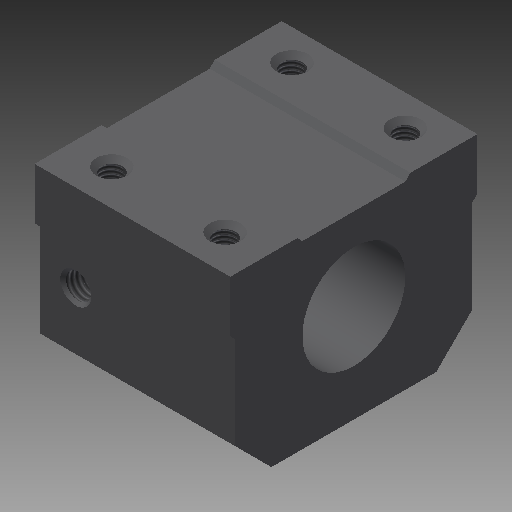
# Autodesk Inventor part: BNT 2010-2.6 Nut
Saved by Autodesk Inventor 2018 (Build 220112000, 112)
## iProperties
Category: PARTsolutions
Company: THK
Created: 2017-05-30
Part Number: BNT 2010-2.6 Nut
Catalog Web Link: www.cadenas.de
Description: BNT Nut-
Vendor: THK
Document SubType Name: Modeling
Designer: psAdmin
Manufacturer: THK
Mass: 82.4787 g
Surface Area: 175.198 cm^2
Volume: 82.4787 cm^3
Density: 1 g/cm^3
Material: Generic
Appearance: PSOLRGB-192-192-192
PSOL_IDENT_0: {$CADENAS_DATA\23d-libs\thk\fed_screw\ball_screw\ball_screw\standard_lead_rbs\bnt\bnt_nut.prj},176 {
PSOL_IDENT_1: VTYP=3D},{NB=BNT 2010-2.6 Nut},{LINA=BNT 2010-2.6 Nut},{NN=BNT Nut},{DATE=16.05.2017 06:09:49},{GEOM
PSOL_IDENT_2: DATE=23.11.2007 13:11:00},{VERSION=},{LINEID=290},{LINESUBID=-1},{WBVAR=}  {NB=BNT 2010-2.6 Nut},{LI
PSOL_IDENT_3: NA=BNT 2010-2.6 Nut},{KT=DUMMY},{MN=BNT 2010-2.6},{L=58.000},{EL=2102.000},{W=48.000},{F=18.000},{B=
PSOL_IDENT_4: 35.000},{C=35.000},{W1=24.000},{T=9.000},{M=46.000},{NDM=6.000},{KDM=4.917},{SL=10.000},{N1=10.000},
PSOL_IDENT_5: {N2=2.000},{A=6.000},{M1=41.400},{X1=1.440},{X2=20.700},{R1=10.170},{X3=4.560},{ANG=47.0},{DK=4.000}
PSOL_IDENT_6: ,{Y=1.770},{X4=0.300},{SD=20},{SL2=10.000},{Y2=14.560}
NN: BNT Nut
NB: BNT 2010-2.6 Nut
NBSYN: $MN. Nut
LINA: BNT 2010-2.6 Nut
MN: BNT 2010-2.6
L: 58.000
EL: 2102.000
W: 48.000
F: 18.000
B: 35.000
C: 35.000
W1: 24.000
T: 9.000
M: 46.000
NDM: 6.000
KDM: 4.917
SL: 10.000
N1: 10.000
N2: 2.000
A: 6.000
M1: 41.400
X1: 1.440
X2: 20.700
R1: 10.170
X3: 4.560
ANG: 47.0
DK: 4.000
Y: 1.770
X4: 0.300
SD: 20
SL2: 10.000
Y2: 14.560
SUPPLIER: THK
ARTICLENO: BNT 2010-2.6 Nut
BOMINFO: BNT 2010-2.6 Nut
CREATOR: CADENAS GmbH
Title: BNT 2010-2.6 Nut
Author: Cadenas PARTsolutions
Autodesk Inventor part; units mm, degrees
ref_plane "YZ Plane" through (0, 0, 0) normal (1, 0, 0) x (0, 1, 0)
ref_plane "XZ Plane" through (0, 0, 0) normal (0, 1, 0) x (-1, 0, 0)
ref_plane "XY Plane" through (0, 0, 0) normal (0, 0, 1) x (1, 0, 0)
sketch "Sketch_1" plane through (0, 0, 0) normal (1, 0, 0) x (0, 1, 0)
  line L0 (17, 24) -> (7, 24)
  line L1 (7, 24) -> (6, 23)
  line L2 (6, 23) -> (-12, 23)
  line L3 (-19, 16) -> (-19, -16)
  line L4 (-12, -23) -> (6, -23)
  line L5 (6, -23) -> (7, -24)
  line L6 (7, -24) -> (17, -24)
  line L7 (17, -24) -> (17, -11)
  line L8 (17, -11) -> (16, -10)
  line L9 (16, -10) -> (16, 10)
  line L10 (16, 10) -> (17, 11)
  line L11 (17, 11) -> (17, 24)
  circle A0 centre (0, 0) radius 10
  line L12 (16, 0) -> (0, 0) construction
  line L13 (-12, -23) -> (-19, -16)
  line L14 (-12, 23) -> (-19, 16)
  line L15 (0, 0) -> (-19, 0) construction
  line L16 (6, 23) -> (6, -23) construction
  dimension "d39" = 20
  dimension "d41" = 46
  dimension "d43" = 23
  dimension "d45" = 1
  dimension "d46" = 48
  dimension "d47" = 1
  dimension "d48" = 36
  dimension "d49" = 10
  dimension "d50" = 10
  dimension "d51" = 20
  dimension "d52" = 13
  dimension "d53" = 13
  dimension "d54" = 32
  dimension "d55" = 16
  dimension "d56" = 135
  dimension "d57" = 18
  dimension "d58" = 18
  constraints: 34 end point, 2 coincident, 2 horizontal, 2 midpoint, 2 parallel, 2 vertical, 1 centre point, 1 collinear, 1 perpendicular, 1 other
  measures "d39" diameter of A0
  measures "d41" distance between parallel lines of L4 L2
  measures "d43" distance from line of L2 L12.end
  measures "d45" distance between parallel lines of L9 L7
  measures "d46" distance between parallel lines of L6 L0
  measures "d47" distance between parallel lines of L4 L6
  measures "d48" distance between parallel lines of L7 L3
  measures "d49" distance of L0.start L0.end
  measures "d50" distance of L5.end L6.end
  measures "d51" distance of L8.end L9.end
  measures "d52" distance of L10.end L0.start
  measures "d53" distance of L6.end L7.end
  measures "d54" distance of L3.start L3.end
  measures "d55" distance from line of L9 L12.end
  measures "d56" angle of L0 L1
  measures "d57" distance of L4.start L4.end
  measures "d58" distance of L1.end L2.end
extrude "Extrusion1" add sketch "Sketch_1" along normal blind 38
sketch "Sketch_2" plane through (29, 0, 0) normal (0.6819984, 0, 0.7313537) x (0.7313537, 0, -0.6819984)
  line L0 (-29, -24.55) -> (-4.4539, -24.55)
  arc A0 (-4.4539, -24.55) -> (4.4539, -24.55) centre (0, -23.4) ccw
  line L1 (4.4539, -24.55) -> (29, -24.55)
  line L2 (29, -24.55) -> (29, -23.4)
  line L3 (29, -23.4) -> (-29, -23.4)
  line L4 (-29, -23.4) -> (-29, -24.55)
  dimension "d33" = 58
  dimension "d34" = 1.15
  dimension "d35" = 24.5461
  dimension "d36" = 4.6
  dimension "d37" = 24.5461
  dimension "d38" = 1.15
  constraints: 10 end point, 2 point on circle, 1 centre point, 1 midpoint, 1 perpendicular
  measures "d33" distance of L2.end L3.end
  measures "d34" distance of L1.end L2.end
  measures "d35" distance of L1.start L1.end
  measures "d36" radius of A0
  measures "d37" distance of L0.start L0.end
  measures "d38" distance of L3.end L0.start
extrude "Extrusion2" [suppressed]
sketch "Sketch_3" plane through (0, -23.4, 0) normal (0, 1, 0) x (1, 0, 0)
  line L0 (-29, -58) -> (87, -58)
  line L1 (87, -58) -> (87, 58)
  line L2 (87, 58) -> (-29, 58)
  line L3 (-29, 58) -> (-29, -58)
  line L4 (9.6667, -9.44) -> (48.3333, -9.44)
  line L5 (48.3333, -9.44) -> (48.3333, 9.44)
  line L6 (48.3333, 9.44) -> (9.6667, 9.44)
  line L7 (9.6667, 9.44) -> (9.6667, -9.44)
  constraints: 16 end point
extrude "Extrusion3" [suppressed]
sketch "Sketch_4" plane through (0, 0, 0) normal (0, 0, 1) x (1, 0, 0)
  line L0 (13.4367, -26.15) -> (13.4367, -24.55)
  line L1 (13.4367, -24.55) -> (15.4367, -24.55)
  line L2 (15.4367, -24.55) -> (15.4367, -25.75)
  arc A0 (15.0367, -26.15) -> (15.4367, -25.75) centre (15.0367, -25.75) ccw
  line L3 (15.0367, -26.15) -> (13.4367, -26.15)
  line L4 (13.4367, -26.15) -> (13.4367, -24.55)
  constraints: 10 end point, 2 point on circle, 1 centre point
revolve "Revolution1" [suppressed]
sketch "Sketch_5" plane through (0, 0, 0) normal (0, 0, 1) x (1, 0, 0)
  line L0 (44.5633, -26.15) -> (44.5633, -24.55)
  line L1 (44.5633, -24.55) -> (46.5633, -24.55)
  line L2 (46.5633, -24.55) -> (46.5633, -25.75)
  arc A0 (46.1633, -26.15) -> (46.5633, -25.75) centre (46.1633, -25.75) ccw
  line L3 (46.1633, -26.15) -> (44.5633, -26.15)
  line L4 (44.5633, -26.15) -> (44.5633, -24.55)
  constraints: 10 end point, 2 point on circle, 1 centre point
revolve "Revolution2" [suppressed]
sketch "Sketch_6" plane through (0, -26.15, 0) normal (0, 1, 0) x (1, 0, 0)
  line L0 (43.5633, 0.15) -> (43.5633, -0.15)
  line L1 (43.5633, -0.15) -> (44.4133, -0.15)
  line L2 (44.4133, -0.15) -> (44.4133, -1)
  line L3 (44.4133, -1) -> (44.7133, -1)
  line L4 (44.7133, -1) -> (44.7133, -0.15)
  line L5 (44.7133, -0.15) -> (45.5633, -0.15)
  line L6 (45.5633, -0.15) -> (45.5633, 0.15)
  line L7 (45.5633, 0.15) -> (44.7133, 0.15)
  line L8 (44.7133, 0.15) -> (44.7133, 1)
  line L9 (44.7133, 1) -> (44.4133, 1)
  line L10 (44.4133, 1) -> (44.4133, 0.15)
  line L11 (44.4133, 0.15) -> (43.5633, 0.15)
  constraints: 24 end point
extrude "Extrusion4" [suppressed]
sketch "Sketch_7" plane through (0, -26.15, 0) normal (0, 1, 0) x (1, 0, 0)
  line L0 (12.4367, 0.15) -> (12.4367, -0.15)
  line L1 (12.4367, -0.15) -> (13.2867, -0.15)
  line L2 (13.2867, -0.15) -> (13.2867, -1)
  line L3 (13.2867, -1) -> (13.5867, -1)
  line L4 (13.5867, -1) -> (13.5867, -0.15)
  line L5 (13.5867, -0.15) -> (14.4367, -0.15)
  line L6 (14.4367, -0.15) -> (14.4367, 0.15)
  line L7 (14.4367, 0.15) -> (13.5867, 0.15)
  line L8 (13.5867, 0.15) -> (13.5867, 1)
  line L9 (13.5867, 1) -> (13.2867, 1)
  line L10 (13.2867, 1) -> (13.2867, 0.15)
  line L11 (13.2867, 0.15) -> (12.4367, 0.15)
  constraints: 24 end point
extrude "Extrusion5" [suppressed]
sketch "Sketch8" plane through (0, -12, 23) normal (0, 0, 1) x (1, 0, 0)
  line L0 (0, 18) -> (0, 0) projected
  point P0 (7, 11.14)
  dimension "d61" = 7
  measures "d61" distance from line of L0 point (7, 11.14)
hole "Hole1" at (7, -0.86, 23) direction (0, 0, -1) diameter 4.917 depth 14.1406 tip angle 120 countersink diameter 6 countersink angle 90 thread size "M6x1" class "6H" standard "ISO Metric profile"
sketch "Sketch9" plane through (0, 17, -11) normal (0, 1, 0) x (1, 0, 0)
  line L0 (0, 13) -> (0, 0) projected
  line L1 (0, 13) -> (38, 13) projected
  point P0 (8, 7)
  dimension "d59" = 8
  dimension "d60" = 6
  measures "d59" distance from line of L0 point (8, 7)
  measures "d60" distance from line of L1 point (8, 7)
hole "Hole2" at (8, 17, -18) direction (0, -1, 0) diameter 4.134 depth 13 tip angle 120 countersink diameter 6 countersink angle 90 thread size "M5x0.8" class "6H" standard "ISO Metric profile"
pattern_linear "Rectangular Pattern1" count 2 spacing 22 along (1, 0, 0) count 2 spacing 35 along (0, 0, 1) of "Hole2"
ref_plane "bnt_nut_1_XY" through (0, 0, 0) normal (1, 0, 0) x (0, 0, -1)
ref_plane "bnt_nut_1_YZ" through (0, 0, 0) normal (0, 0, -1) x (0, 1, 0)
ref_plane "bnt_nut_1_ZX" through (0, 0, 0) normal (0, 1, 0) x (1, 0, 0)
sketch "Sketch10" plane through (38, -23.4, -9.44) normal (0, 0, -1) x (-1, 0, 0)
  point P0 (38, 23.4)
sketch "Sketch11" plane through (38, 0, 0) normal (1, 0, 0) x (0, 0, -1)
  circle A0 centre (0, 0) radius 15.5
  dimension "d62" = 31
  constraints: 1 centre point, 1 coincident
  measures "d62" diameter of A0
body "Solid1"
